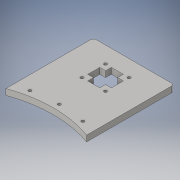
# Autodesk Inventor part: Camera_Mount_Acryllic
Saved by Autodesk Inventor 2016 (Build 200138000, 138)
## iProperties
Created: 2016-04-19
Part Number: Camera_Mount_Acryllic
Material: Generic
Document SubType Name: Modeling
Designer: Ethan
Density: 1 g/cm^3
Appearance: Default
Author: Ethan
Autodesk Inventor part; units mm, degrees
ref_plane "YZ Plane" through (0, 0, 0) normal (1, 0, 0) x (0, 1, 0)
ref_plane "XZ Plane" through (0, 0, 0) normal (0, 1, 0) x (-1, 0, 0)
ref_plane "XY Plane" through (0, 0, 0) normal (0, 0, 1) x (1, 0, 0)
sketch "Sketch1" plane through (0, 0, 0) normal (0, 1, 0) x (-1, 0, 0)
  circle A0 centre (0, -133.35) radius 1.5875
  line L0 (1.5875, -133.35) -> (-1.5875, -133.35)
  line L1 (-42.8213, -132.9753) -> (-42.8213, -119.5631)
  line L2 (-6.4213, -188.8018) -> (-12.5713, -188.8018)
  line L3 (-6.4213, -194.9518) -> (-6.4213, -188.8018)
  line L4 (-12.5713, -188.8018) -> (-12.5713, -176.1018)
  line L5 (-12.5713, -188.8018) -> (-12.5713, -176.1018)
  line L6 (6.2787, -194.9518) -> (-6.4213, -194.9518)
  line L7 (6.2787, -194.9518) -> (-6.4213, -194.9518)
  line L8 (-12.5713, -176.1018) -> (-6.4213, -176.1018)
  line L9 (6.2787, -188.8018) -> (6.2787, -194.9518)
  line L10 (-6.4213, -176.1018) -> (-6.4213, -169.9518)
  line L11 (-6.4213, -194.9518) -> (-6.4213, -169.9518)
  line L12 (6.2787, -169.9518) -> (6.2787, -194.9518)
  line L13 (-6.4213, -169.9518) -> (6.2787, -169.9518)
  line L14 (-6.4213, -169.9518) -> (6.2787, -169.9518)
  line L15 (-12.5713, -176.1018) -> (12.4167, -176.1018)
  line L16 (12.4167, -188.8018) -> (-12.5713, -188.8018)
  circle A1 centre (-12.5713, -194.9518) radius 1.5875
  line L17 (6.2787, -169.9518) -> (6.2787, -176.1018)
  line L18 (12.4167, -188.8018) -> (6.2787, -188.8018)
  line L19 (6.2787, -176.1018) -> (12.4167, -176.1018)
  line L20 (12.4167, -176.1018) -> (12.4167, -188.8018)
  line L21 (12.4167, -176.1018) -> (12.4167, -188.8018)
  line L22 (0, -169.5003) -> (0, -169.4888)
  circle A2 centre (12.4287, -169.9518) radius 1.5875
  circle A3 centre (-12.5713, -169.9518) radius 1.5875
  circle A4 centre (12.4287, -194.9518) radius 1.5875
  circle A5 centre (-28.1555, -130.3624) radius 1.5875
  line L23 (0, -131.7625) -> (0, -134.9375)
  line L24 (-42.8213, -119.5631) -> (42.8213, -119.5631)
  line L25 (42.8213, -119.5631) -> (42.8213, -209.2768)
  line L26 (39.6463, -212.4518) -> (-39.6463, -212.4518)
  line L27 (-42.8213, -209.2768) -> (-42.8213, -119.5631)
  circle A6 centre (28.1555, -130.3624) radius 1.5875
  arc A7 (39.6463, -212.4518) -> (42.8213, -209.2768) centre (39.6463, -209.2768) ccw
  arc A8 (-42.8213, -209.2768) -> (-39.6463, -212.4518) centre (-39.6463, -209.2768) ccw
  arc A9 (-42.8213, -119.5631) -> (42.8213, -119.5631) centre (0, 0) ccw
  point P0 (-26.811, -129.5183)
  point P1 (-26.811, -129.5183)
  point P2 (26.811, -129.5183)
  point P3 (26.811, -129.5183)
  dimension "d0" = 3.175
  dimension "d2" = 36.6018
  dimension "d4" = 25
  dimension "d6" = 3.175
  dimension "d8" = 3.175
  dimension "d9" = 254
  constraints: 56 end point, 14 point on circle, 10 centre point, 4 tangent, 3 coincident, 3 symmetric about line, 2 horizontal, 2 parallel, 1 equal radius, 1 perpendicular, 1 vertical, 5 other
  measures "d0" diameter of A0
  measures "d2" vertical distance of A0.centre A3.centre
  measures "d4" distance of A3.centre A2.centre
  measures "d6" diameter of A5
  measures "d8" radius of A7
  measures "d9" diameter of A9
extrude "Extrusion1" add sketch "Sketch1" along normal blind 6.35 contours L1 A9 L25 A7 L26 A8 L27
body "Solid1"
